Autodesk Fusion 360 part; units mm, degrees
(part 24 of 24)
sketch "Sketch1" plane through (0, 0, 0) normal (0, 1, 0) x (1, 0, 0)
  line L0 (0, 0) -> (30, 0)
  line L1 (30, 0) -> (30, -27)
  line L2 (30, -27) -> (0, -27)
  line L3 (0, -27) -> (0, 0)
  line L4 (6.5, -27) -> (6.5, -25)
  line L5 (6.5, -25) -> (23.5, -25)
  line L6 (23.5, -25) -> (23.5, -27)
  line L7 (15, -27) -> (15, -25) construction
  line L8 (3.5, -4.3) -> (26.5, -4.3)
  line L9 (26.5, -4.3) -> (26.5, -22.7)
  line L10 (26.5, -22.7) -> (3.5, -22.7)
  line L11 (3.5, -22.7) -> (3.5, -4.3)
  line L12 (1.5, -2.5) -> (4, -2.5)
  arc A0 (4, -2.5) -> (4, -0.5) centre (4, -1.5) ccw
  line L13 (4, -0.5) -> (1.5, -0.5)
  arc A1 (1.5, -0.5) -> (1.5, -2.5) centre (1.5, -1.5) ccw
  line L14 (1.5, -1.5) -> (4, -1.5) construction
  line L15 (15, 0) -> (15, -25) construction
  line L16 (0, -13.5) -> (30, -13.5) construction
  arc A2 (26, -0.5) -> (26, -2.5) centre (26, -1.5) ccw
  line L17 (26, -0.5) -> (28.5, -0.5)
  arc A3 (28.5, -2.5) -> (28.5, -0.5) centre (28.5, -1.5) ccw
  line L18 (28.5, -2.5) -> (26, -2.5)
  line L19 (26, -26.5) -> (28.5, -26.5)
  arc A4 (28.5, -26.5) -> (28.5, -24.5) centre (28.5, -25.5) ccw
  line L20 (28.5, -24.5) -> (26, -24.5)
  arc A5 (26, -24.5) -> (26, -26.5) centre (26, -25.5) ccw
  line L21 (4, -26.5) -> (1.5, -26.5)
  arc A6 (4, -26.5) -> (4, -24.5) centre (4, -25.5) ccw
  arc A7 (1.5, -24.5) -> (1.5, -26.5) centre (1.5, -25.5) ccw
  line L22 (1.5, -24.5) -> (4, -24.5)
  dimension "d1" = 30
  dimension "d2" = 27
  dimension "d3" = 6.5
  dimension "d4" = 2
  dimension "d5" = 3.5
  dimension "d6" = 3.5
  dimension "d7" = 4.3
  dimension "d8" = 4.3
  dimension "d22" = 1.5
  dimension "d23" = 1.5
  dimension "d24" = 1
  dimension "d25" = 2.5
  constraint horizontal L0
  constraint vertical L1
  constraint horizontal L2
  constraint vertical L3
  constraint coincident L0.start L3.end
  constraint coincident L2 L4.start
  constraint perpendicular L2 L4
  constraint perpendicular L4 L5
  constraint coincident L2 L6.end
  constraint perpendicular L2 L6
  constraint midpoint L2 L7.start
  constraint midpoint L5 L7.end
  constraint perpendicular L2 L7
  constraint horizontal L8
  constraint vertical L9
  constraint horizontal L10
  constraint vertical L11
  constraint tangent L12 A0
  constraint tangent A0 L13
  constraint parallel L12 L13
  constraint tangent L13 A1
  constraint tangent L12 A1
  constraint horizontal L14
  constraint midpoint L0 L15.start
  constraint midpoint L3 L16.start
  constraint midpoint L1 L16.end
  constraint symmetric L12.start L15 A3.start
  constraint symmetric L12.end L15 A2.end
  constraint symmetric A0.end L15 A2.start
  constraint symmetric L13.end L15 L17.end
  constraint symmetric A0 L15 A2
  constraint symmetric A1 L15 A3
  constraint symmetric L12.start L16 A7.start
  constraint symmetric L12.end L16 A6.end
  constraint symmetric A0.end L16 L21.start
  constraint symmetric L13.end L16 L21.end
  constraint symmetric A0 L16 A6
  constraint symmetric A1 L16 A7
  constraint symmetric L16 A2.end L20.end
  constraint symmetric L16 A2.start L19.start
  constraint symmetric L16 A2 A5
  constraint symmetric L16 L17.end L19.end
  constraint symmetric L16 A3.start A4.end
  constraint symmetric L16 A3 A4
  measures "d1" distance of L0.start L0.end
  measures "d2" distance of L0.start L2.end
  measures "d3" distance of L1 L6
  measures "d4" distance of L2 L5
  measures "d5" distance of L1 L9
  measures "d6" distance of L3 L11
  measures "d7" distance of L0 L8
  measures "d8" distance of L2 L10
  measures "d22" distance of L3 A1.centre
  measures "d23" distance of L0 A1.centre
  measures "d24" radius of A1
  measures "d25" distance of A1.centre A0.centre
extrude "Extrude1" add sketch "Sketch1" along normal blind 1 contours L8 L9 L10 L11 makes body 1
extrude "Extrude2" add sketch "Sketch1" against normal blind 1 separate body contours L0 L1 L2 L3 L4 L5 L6 | L8 L9 L10 L11 makes body 2
sketch "Sketch2" plane through (0, -1, 0) normal (0, -1, 0) x (1, 0, 0)
  line L0 (6.5, 25) -> (6.5, 27)
  line L1 (6.5, 27) -> (0, 27)
  line L2 (0, 27) -> (0, 0)
  line L3 (0, 0) -> (30, 0)
  line L4 (30, 0) -> (30, 27)
  line L5 (30, 27) -> (23.5, 27)
  line L6 (23.5, 27) -> (23.5, 25)
  line L7 (23.5, 25) -> (6.5, 25)
  line L8 (10.1, 2.6) -> (19.9, 2.6)
  line L9 (19.9, 2.6) -> (19.9, 0)
  line L10 (10.1, 0) -> (10.1, 2.6)
  line L11 (15, 0) -> (15, 2.6) construction
  arc A0 (26, 2.5) -> (26, 0.5) centre (26, 1.5) ccw
  line L12 (26, 2.5) -> (28.5, 2.5)
  arc A1 (28.5, 0.5) -> (28.5, 2.5) centre (28.5, 1.5) ccw
  line L13 (28.5, 0.5) -> (26, 0.5)
  arc A2 (26, 26.5) -> (26, 24.5) centre (26, 25.5) ccw
  line L14 (26, 26.5) -> (28.5, 26.5)
  arc A3 (28.5, 24.5) -> (28.5, 26.5) centre (28.5, 25.5) ccw
  line L15 (28.5, 24.5) -> (26, 24.5)
  arc A4 (4, 24.5) -> (4, 26.5) centre (4, 25.5) ccw
  line L16 (4, 24.5) -> (1.5, 24.5)
  arc A5 (1.5, 26.5) -> (1.5, 24.5) centre (1.5, 25.5) ccw
  line L17 (1.5, 26.5) -> (4, 26.5)
  arc A6 (1.5, 2.5) -> (1.5, 0.5) centre (1.5, 1.5) ccw
  line L18 (1.5, 2.5) -> (4, 2.5)
  arc A7 (4, 0.5) -> (4, 2.5) centre (4, 1.5) ccw
  line L19 (4, 0.5) -> (1.5, 0.5)
  dimension "d13" = 9.8
  dimension "d14" = 2.6
  constraint horizontal L8
  constraint vertical L9
  constraint vertical L10
  constraint midpoint L3 L11.start
  constraint perpendicular L3 L11
  constraint coincident L3 L9.end
  constraint coincident L3 L10.start
  constraint midpoint L8 L11.end
  measures "d13" distance of L8.start L8.end
  measures "d14" distance of L8.start L10.start
extrude "Extrude3" add sketch "Sketch2" along normal blind 15 separate body contours L3 L8 L9 L10 makes body 3
sketch "Minimal Projection" plane through (0, -1, 0) normal (0, -1, 0) x (1, 0, 0)
  arc A0 (26, 2.5) -> (26, 0.5) centre (26, 1.5) ccw
  line L0 (26, 2.5) -> (28.5, 2.5)
  arc A1 (28.5, 0.5) -> (28.5, 2.5) centre (28.5, 1.5) ccw
  line L1 (28.5, 0.5) -> (26, 0.5)
  arc A2 (26, 26.5) -> (26, 24.5) centre (26, 25.5) ccw
  line L2 (26, 26.5) -> (28.5, 26.5)
  arc A3 (28.5, 24.5) -> (28.5, 26.5) centre (28.5, 25.5) ccw
  line L3 (28.5, 24.5) -> (26, 24.5)
  arc A4 (4, 24.5) -> (4, 26.5) centre (4, 25.5) ccw
  line L4 (4, 24.5) -> (1.5, 24.5)
  arc A5 (1.5, 26.5) -> (1.5, 24.5) centre (1.5, 25.5) ccw
  line L5 (1.5, 26.5) -> (4, 26.5)
  arc A6 (1.5, 2.5) -> (1.5, 0.5) centre (1.5, 1.5) ccw
  line L6 (1.5, 2.5) -> (4, 2.5)
  arc A7 (4, 0.5) -> (4, 2.5) centre (4, 1.5) ccw
  line L7 (4, 0.5) -> (1.5, 0.5)
  line L8 (6.5, 25) -> (6.5, 27)
  line L9 (6.5, 27) -> (0, 27)
  line L10 (0, 27) -> (0, 0)
  line L11 (0, 0) -> (30, 0)
  line L12 (30, 0) -> (30, 27)
  line L13 (30, 27) -> (23.5, 27)
  line L14 (23.5, 27) -> (23.5, 25)
  line L15 (23.5, 25) -> (6.5, 25)
  line L16 (19.9, 0) -> (19.9, 2.6)
  line L17 (19.9, 2.6) -> (10.1, 2.6)
  line L18 (10.1, 2.6) -> (10.1, 0)
